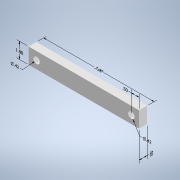
# Autodesk Inventor part: connectingRod-4-in
Saved by Autodesk Inventor 2020.2 (Build 242310000, 310)
## iProperties
Created: 2020-01-13
Part Number: connectingRod-4-in
Material: Generic
Document SubType Name: Modeling
Designer: robst
Density: 1 g/cm^3
Appearance: Default
Author: robst
Autodesk Inventor part; units mm, degrees
ref_plane "YZ Plane" through (0, 0, 0) normal (1, 0, 0) x (0, 1, 0)
ref_plane "XZ Plane" through (0, 0, 0) normal (0, 1, 0) x (-1, 0, 0)
ref_plane "XY Plane" through (0, 0, 0) normal (0, 0, 1) x (1, 0, 0)
sketch "Sketch1" plane through (0, 0, 0) normal (0, 0, 1) x (1, 0, 0)
  line L0 (-88.9, 12.7) -> (88.9, 12.7)
  line L1 (88.9, 12.7) -> (88.9, -12.7)
  line L2 (88.9, -12.7) -> (-88.9, -12.7)
  line L3 (-88.9, -12.7) -> (-88.9, 12.7)
  line L4 (-88.9, 12.7) -> (88.9, -12.7) construction
  line L5 (88.9, 12.7) -> (-88.9, -12.7) construction
  circle A0 centre (-76.2, 0) radius 5.2705
  circle A1 centre (76.2, 0) radius 5.2705
  point P0 (0, 0)
  dimension "d0" = 177.8
  dimension "d1" = 25.4
  dimension "d2" = 10.541
  dimension "d3" = 12.7
  dimension "d5" = 12.7
  constraints: 12 end point, 2 centre point, 2 midpoint, 2 parallel, 1 equal radius, 1 horizontal, 1 perpendicular
  measures "d0" distance of L1.end L2.end
  measures "d1" distance of L0.end L1.end
  measures "d2" diameter of A0
  measures "d3" distance from line of A0.centre L3
  measures "d5" distance from line of A1.centre L1
extrude "Extrusion1" add sketch "Sketch1" along normal mid plane 12.7
body "Solid1"
